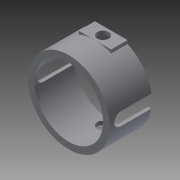
# Autodesk Inventor part: optoforce_base
Saved by Autodesk Inventor 2015 (Build 190159000, 159)
## iProperties
Created: 2015-09-26
Part Number: optoforce_base
Material: Générique
Document SubType Name: Modeling
Designer: astralien3000
Density: 1 g/cm^3
Appearance: Par défaut
Author: astralien3000
Autodesk Inventor part; units mm, degrees
ref_plane "YZ Plane" through (0, 0, 0) normal (1, 0, 0) x (0, 1, 0)
ref_plane "XZ Plane" through (0, 0, 0) normal (0, 1, 0) x (-1, 0, 0)
ref_plane "XY Plane" through (0, 0, 0) normal (0, 0, 1) x (1, 0, 0)
sketch "Esquisse1" plane through (0, 0, 0) normal (0, 1, 0) x (-1, 0, 0)
  circle A0 centre (0, 0) radius 10.5
  circle A1 centre (0, 0) radius 12.5
  dimension "d0" = 21
  dimension "d1" = 25
  constraints: 2 centre point, 2 coincident
  measures "d0" diameter of A0
  measures "d1" diameter of A1
extrude "Extrusion1" add sketch "Esquisse1" along normal blind 1
sketch "Esquisse2" plane through (0, 1, 0) normal (0, 1, 0) x (1, 0, 0)
  circle A0 centre (0, 0) radius 12.5
  circle A1 centre (0, 0) radius 11.5
  dimension "d4" = 23
  dimension "d5" = 25
  constraints: 2 centre point, 2 coincident
  measures "d4" diameter of A1
  measures "d5" diameter of A0
extrude "Extrusion2" add sketch "Esquisse2" along normal blind 12
sketch "Esquisse3" plane through (0, 13, 0) normal (0, 1, 0) x (1, 0, 0)
  line L0 (-5, -12.5) -> (5, -12.5)
  line L1 (5, -12.5) -> (5, -10.3562)
  line L2 (5, 12.5) -> (-5, 12.5)
  line L3 (-5, 12.5) -> (-5, 10.3562)
  circle A0 centre (0, 0) radius 12.5 projected
  arc A1 (-5, 10.3562) -> (-5, -10.3562) centre (0, 0) ccw
  circle A2 centre (0, 0) radius 11.5 projected
  arc A3 (5, 10.3562) -> (-5, 10.3562) centre (0, 0) ccw
  arc A4 (-5, -10.3562) -> (5, -10.3562) centre (0, 0) ccw
  arc A5 (5, -10.3562) -> (5, 10.3562) centre (0, 0) ccw
  line L4 (-5, 10.3562) -> (-5, -10.3562)
  line L5 (-5, -10.3562) -> (-5, -12.5)
  line L6 (5, 10.3562) -> (5, 12.5)
  line L7 (5, -10.3562) -> (5, 10.3562)
  dimension "d8" = 5
  dimension "d9" = 5
  dimension "d10" = 0
  constraints: 16 end point, 10 parallel, 8 point on circle, 4 centre point, 3 perpendicular, 2 tangent, 1 coincident, 1 horizontal, 1 point on line
  measures "d8" distance from line of point (0, 0) L3
  measures "d9" distance from line of L1 point (0, 0)
  measures "d10" radial gap between concentric circles of A2 A1
extrude "Extrusion3" add sketch "Esquisse3" against normal blind 5 contours L5 A0 L0 | A0 L1 L0 | A0 L5 A2 L1 | A0 L6 A2 L3 | L3 L2 A0 | L2 L6 A0
sketch "Esquisse4" plane through (-5, 13, 12.5) normal (0, 0, 1) x (1, 0, 0)
  line L0 (10, -5) -> (0, 0) construction
  line L1 (10, 0) -> (0, -5) construction
  circle A0 centre (5, -2.5) radius 1.75
  point P0 (5, -13)
  dimension "d13" = 3.5
  constraints: 4 end point, 1 centre point, 1 midpoint
  measures "d13" diameter of A0
extrude "Extrusion4" cut sketch "Esquisse4" against normal through all
sketch "Esquisse6" plane through (0, 13, 0) normal (0, 1, 0) x (1, 0, 0)
  line L0 (-12.5, -2) -> (12.5, -2)
  line L1 (12.5, -2) -> (12.5, 2)
  line L2 (12.5, 2) -> (-12.5, 2)
  line L3 (-12.5, 2) -> (-12.5, -2)
  arc A0 (-5, 11.4564) -> (-5, -11.4564) centre (0, 0) ccw projected
  arc A1 (5, -11.4564) -> (5, 11.4564) centre (0, 0) ccw projected
  dimension "d17" = 4
  dimension "d18" = 2
  constraints: 8 end point, 2 parallel, 2 tangent, 1 horizontal, 1 perpendicular
  measures "d17" distance between parallel lines of L0 L2
  measures "d18" distance from line of A0.centre L2
extrude "Extrusion5" cut sketch "Esquisse6" against normal blind 9.5
sketch "Esquisse7" plane through (0, 3.5, 0) normal (0, 1, 0) x (1, 0, 0)
  line L0 (-12.5, -2) -> (12.5, -2)
  line L1 (12.5, -2) -> (12.5, 0)
  line L2 (12.5, 2) -> (-12.5, 2)
  line L3 (-12.5, 2) -> (-12.5, 0)
  line L4 (-11.3248, -2) -> (-12.339, -2) projected
  line L5 (-12.339, 2) -> (-11.3248, 2) projected
  arc A0 (-12.339, 2) -> (-12.339, -2) centre (0, 0) ccw projected
  arc A1 (12.339, -2) -> (12.339, 2) centre (0, 0) ccw projected
  line L6 (-12.5, 0) -> (12.5, 0)
  line L7 (-12.5, 0) -> (-12.5, -2)
  line L8 (12.5, 0) -> (12.5, 2)
  constraints: 14 end point, 5 parallel, 4 tangent, 2 collinear, 2 perpendicular, 2 point on circle, 1 horizontal
revolve "Révolution1" cut sketch "Esquisse7" angle 360 about axis through (-12.5, 3.5, 0) along (1, 0, 0) contours L3 L2 A0 | A0 L2 A1 L6 | A1 L2 L8
equation "\"d18\" = 0.5 * d17"
